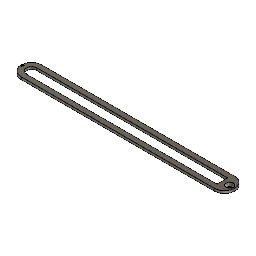
_Sharpie Line Maker 2000.1d570de3-5c31-4fa7-a778-c33d8cc0cd13 (Autodesk Fusion 360 design; units mm, degrees)
Autodesk Fusion 360 part; units mm, degrees
sketch "Sketch1" plane through (0, 0, 0) normal (0, 0, 1) x (1, 0, 0)
  line L0 (0, 0) -> (0, -12.7)
  line L1 (12.7, 0) -> (254, 0)
  line L2 (254, -25.4) -> (12.7, -25.4)
  line L3 (0, -25.4) -> (0, -12.7)
  arc A0 (12.7, 0) -> (0, -12.7) centre (12.7, -12.7) ccw
  arc A1 (0, -12.7) -> (12.7, -25.4) centre (12.7, -12.7) ccw
  circle A2 centre (254, -12.7) radius 1.27
  line L4 (254, -25.4) -> (255.27, -25.4)
  line L5 (255.27, 0) -> (254, 0)
  line L6 (255.27, 0) -> (245.11, 0)
  line L7 (245.11, -25.4) -> (255.27, -25.4)
  arc A3 (257.81, -12.7) -> (245.11, 0) centre (245.11, -12.7) ccw
  arc A4 (245.11, -25.4) -> (257.81, -12.7) centre (245.11, -12.7) ccw
  arc A5 (245.11, -19.05) -> (251.46, -12.7) centre (245.11, -12.7) ccw
  arc A6 (251.46, -12.7) -> (245.11, -6.35) centre (245.11, -12.7) ccw
  line L8 (254, -19.05) -> (12.7, -19.05)
  line L9 (12.7, -6.35) -> (254, -6.35)
  arc A7 (12.7, -6.35) -> (6.35, -12.7) centre (12.7, -12.7) ccw
  arc A8 (6.35, -12.7) -> (12.7, -19.05) centre (12.7, -12.7) ccw
  point P0 (0, -25.4)
  point P1 (257.81, 0)
  dimension "d1" = 25.4
  dimension "d3" = 12.7
  dimension "d4" = 12.7
  dimension "d5" = 2.54
  dimension "d6" = 2.54
  dimension "d7" = 12.7
  dimension "d8" = 12.7
  dimension "d9" = -6.35
  dimension "d10" = 6.35
  dimension "d11" = 6.35
  dimension "d12" = -6.35
  constraint coincident L0.start origin
  constraint vertical L0
  constraint horizontal L1
  constraint horizontal L2
  constraint vertical L3
  constraint coincident L0.start L1
  constraint coincident L0.start L3
  constraint tangent L1 A0
  constraint tangent L3 A0
  constraint coincident P0 L2
  constraint coincident P0 L0
  constraint tangent L2 A1
  constraint tangent L0 A1
  constraint horizontal L4
  constraint horizontal L5
  constraint horizontal L6
  constraint horizontal L7
  constraint coincident P1 L6
  constraint tangent L6 A3
  constraint tangent L7 A4
  constraint coincident A3.start A4.end
  measures "d1" distance of L0.start P0
  measures "d3" radius of A0
  measures "d4" radius of A1
  measures "d5" diameter of A2
  measures "d6" distance of L5.start P1
  measures "d7" radius of A3
  measures "d8" radius of A4
extrude "Extrude1" add sketch "Sketch1" along normal blind 3.175
sketch "Sketch2" plane through (0, 0, 3.175) normal (0, 0, 1) x (-1, 0, 0)
  circle A0 centre (-254, 12.7) radius 1.27
  arc A1 (-12.7, 6.35) -> (-12.7, 19.05) centre (-12.7, 12.7) ccw
  line L0 (-12.7, 6.35) -> (-245.11, 6.35)
  arc A2 (-245.11, 19.05) -> (-245.11, 6.35) centre (-245.11, 12.7) ccw
  line L1 (-245.11, 19.05) -> (-12.7, 19.05)
  arc A3 (-12.7, 0) -> (-12.7, 25.4) centre (-12.7, 12.7) ccw
  line L2 (-12.7, 25.4) -> (-245.11, 25.4)
  arc A4 (-245.11, 25.4) -> (-245.11, 0) centre (-245.11, 12.7) ccw
  line L3 (-245.11, 0) -> (-12.7, 0)
  circle A5 centre (-254, 12.7) radius 2.0476
  constraint concentric A0 A5
extrude "Extrude2" cut sketch "Sketch2" against normal blind 2.54 contours A5
sketch "Sketch3" plane through (0, 0, 3.175) normal (0, 0, 1) x (-1, 0, 0)
  circle A0 centre (-254, 12.7) radius 2.0476
  arc A1 (-12.7, 6.35) -> (-12.7, 19.05) centre (-12.7, 12.7) ccw
  line L0 (-12.7, 6.35) -> (-245.11, 6.35)
  line L1 (-245.11, 19.05) -> (-12.7, 19.05)
  arc A2 (-12.7, 0) -> (-12.7, 25.4) centre (-12.7, 12.7) ccw
  line L2 (-12.7, 25.4) -> (-245.11, 25.4)
  arc A3 (-245.11, 25.4) -> (-245.11, 0) centre (-245.11, 12.7) ccw
  line L3 (-245.11, 0) -> (-12.7, 0)
  line L4 (-245.11, 6.35) -> (-251.46, 6.35)
  line L5 (-251.46, 6.35) -> (-251.46, 19.05)
  line L6 (-251.46, 19.05) -> (-245.11, 19.05)
  line L7 (-245.11, 19.05) -> (-245.11, 6.35)
  constraint horizontal L4
  constraint vertical L5
  constraint horizontal L6
  constraint vertical L7
  constraint coincident L0.end L4.start
extrude "Extrude3" add sketch "Sketch3" against normal blind 3.175 contours L4 L5 L6 L7
sketch "Sketch4" plane through (0, 0, 3.175) normal (0, 0, 1) x (-1, 0, 0)
  arc A0 (-12.7, 0) -> (-12.7, 25.4) centre (-12.7, 12.7) ccw
  line L0 (-12.7, 25.4) -> (-245.11, 25.4)
  arc A1 (-245.11, 25.4) -> (-245.11, 0) centre (-245.11, 12.7) ccw
  line L1 (-245.11, 0) -> (-12.7, 0)
  circle A2 centre (-254, 12.7) radius 2.0476
  line L2 (-245.11, 19.05) -> (-12.7, 19.05)
  arc A3 (-12.7, 6.35) -> (-12.7, 19.05) centre (-12.7, 12.7) ccw
  line L3 (-12.7, 6.35) -> (-245.11, 6.35)
  line L4 (-245.11, 6.35) -> (-245.11, 19.05)
  line L5 (-245.11, 0) -> (-260.3587, 0)
  line L6 (-260.3587, 0) -> (-260.3587, 25.4)
  line L7 (-260.3587, 25.4) -> (-245.11, 25.4)
  line L8 (-245.11, 25.4) -> (-245.11, 0)
  constraint horizontal L5
  constraint vertical L6
  constraint horizontal L7
  constraint vertical L8
  constraint coincident A1.end L1.start
extrude "Extrude4" add sketch "Sketch4" against normal blind 3.175 contours A1 L5 L6 L7
extrude "Extrude5" cut 1 faces at (254.0316, -14.4834, 0.635) along direction (0, 0, -1) blind 0.3175
draft "Draft1" angle 40 neutral plane through (0, 0, 0.3175) pull (0, 0, 1) 1 faces at (253.949, -14.747, 2.2225)
fillet "Fillet1" radius 12.7 1 edges at (260.3587, -25.4, 1.5875)
fillet "Fillet2" radius 12.7 1 edges at (260.3587, 0, 1.5875)
sketch "Sketch5" plane through (0, 0, 3.175) normal (0, 0, 1) x (-1, 0, 0)
  arc A0 (-247.6587, 25.4) -> (-247.6587, 0) centre (-247.6587, 12.7) ccw
  line L0 (-247.6587, 0) -> (-12.7, 0)
  arc A1 (-12.7, 0) -> (-12.7, 25.4) centre (-12.7, 12.7) ccw
  line L1 (-12.7, 25.4) -> (-247.6587, 25.4)
  line L2 (-245.11, 19.05) -> (-12.7, 19.05)
  arc A2 (-12.7, 6.35) -> (-12.7, 19.05) centre (-12.7, 12.7) ccw
  line L3 (-12.7, 6.35) -> (-245.11, 6.35)
  line L4 (-245.11, 6.35) -> (-245.11, 19.05)
  circle A3 centre (-254, 12.7) radius 4.4453
  line L5 (0, 12.7) -> (-6.35, 12.7)
  line L6 (-0.1678, 12.7) -> (-1.016, 11.938)
  line L7 (-1.016, 11.938) -> (-1.988, 11.0648)
  line L8 (-0.1678, 12.7) -> (-1.016, 13.462)
  line L9 (-1.016, 13.462) -> (-1.988, 14.3352)
  line L10 (-1.988, 11.0648) -> (-1.988, 14.3352)
  constraint midpoint A1 L5.start
  constraint midpoint A2 L5.end
  constraint coincident L5 L6.start
  constraint symmetric L5 L6.start L8.start
  constraint symmetric L5 L6.end L8.end
  constraint symmetric L5 L7.end L9.end
extrude "Extrude6" cut sketch "Sketch5" against normal blind 0.508 contours L5 L6 L7 L10 | L5 L8 L9 L10
equation "d21 = ( -0.025 / 2 ) * 1 in"
